Autodesk Fusion 360 part; units mm, degrees
note: some values were not read from the file. Set by a fixed rule: which sketch regions a step uses.
(part 2 of 2)
  spline S166 degree 3 poles (44.496223, -52.511943) (44.032677, -52.733983) (43.546131, -52.910026) (43.0817, -53.132067) knots 0 0 0 0 1 1 1 1
  spline S167 degree 3 poles (43.0817, -53.132067) (42.433267, -53.440805) (41.829948, -53.807926) (41.141706, -54.029969) knots 0 0 0 0 1 1 1 1
  spline S168 degree 3 poles (41.141706, -54.029969) (40.538388, -54.224586) (39.320253, -54.821711) (38.725781, -54.625323) knots 0 0 0 0 1 1 1 1
  spline S169 degree 3 poles (38.725781, -54.625323) (38.425005, -54.526245) (38.187042, -54.275896) (38.151654, -53.951235) knots 0 0 0 0 1 1 1 1
  spline S170 degree 3 poles (38.151654, -53.951235) (38.101232, -53.494766) (38.35335, -53.069259) (38.402889, -52.62429) knots 0 0 0 0 1 1 1 1
  spline S171 degree 3 poles (38.402889, -52.62429) (38.444467, -52.258052) (38.431198, -51.852892) (38.384312, -51.487539) knots 0 0 0 0 1 1 1 1
  spline S172 degree 3 poles (38.384312, -51.487539) (38.315311, -50.945261) (38.092385, -50.324251) (38.721356, -50.009323) knots 0 0 0 0 1 1 1 1
  spline S173 degree 3 poles (38.721356, -50.009323) (40.090765, -49.322849) (40.129689, -51.914817) (40.06511, -52.62429) knots 0 0 0 0 1 1 1 1
  spline S174 degree 3 poles (3.607727, -48.243602) (4.740053, -47.180274) (5.990036, -46.481417) (7.50983, -46.140834) knots 0 0 0 0 1 1 1 1
  spline S175 degree 3 poles (7.50983, -46.140834) (8.096341, -46.00991) (8.691695, -45.924101) (9.292362, -45.897561) knots 0 0 0 0 1 1 1 1
  spline S176 degree 3 poles (9.292362, -45.897561) (9.454251, -45.889599) (9.613484, -45.942678) (9.774487, -45.911715) knots 0 0 0 0 1 1 1 1
  spline S177 degree 3 poles (9.774487, -45.911715) (10.134532, -45.842714) (10.56269, -45.601209) (10.90062, -45.453477) knots 0 0 0 0 1 1 1 1
  spline S178 degree 3 poles (10.90062, -45.453477) (11.100547, -45.366782) (11.265972, -45.223473) (11.45705, -45.120855) knots 0 0 0 0 1 1 1 1
  spline S179 degree 3 poles (11.45705, -45.120855) (12.492954, -44.563539) (13.561589, -44.033647) (14.614296, -43.507291) knots 0 0 0 0 1 1 1 1
  spline S180 degree 3 poles (14.614296, -43.507291) (16.420715, -42.602313) (18.244822, -41.723876) (20.039735, -40.791474) knots 0 0 0 0 1 1 1 1
  spline S181 degree 3 poles (20.039735, -40.791474) (20.539553, -40.531393) (21.011057, -40.22089) (21.513526, -39.967884) knots 0 0 0 0 1 1 1 1
  spline S182 degree 3 poles (21.513526, -39.967884) (23.597715, -38.917828) (25.688097, -37.874851) (27.798829, -36.8761) knots 0 0 0 0 1 1 1 1
  spline S183 degree 3 poles (27.798829, -36.8761) (28.349066, -36.616018) (28.951499, -36.454135) (29.485819, -36.170167) knots 0 0 0 0 1 1 1 1
  spline S184 degree 3 poles (29.485819, -36.170167) (29.45574, -35.344805) (29.262891, -34.507063) (29.145234, -33.690546) knots 0 0 0 0 1 1 1 1
  spline S185 degree 3 poles (29.145234, -33.690546) (29.062964, -33.119078) (29.078886, -32.501608) (29.055, -31.923941) knots 0 0 0 0 1 1 1 1
  spline S186 degree 3 poles (29.055, -31.923941) (29.030233, -31.341853) (29.185928, -30.081255) (28.996616, -29.618595) knots 0 0 0 0 1 1 1 1
  spline S187 degree 3 poles (28.996616, -29.618595) (28.600304, -29.789328) (28.245566, -30.021986) (27.865176, -30.221028) knots 0 0 0 0 1 1 1 1
  spline S188 degree 3 poles (27.865176, -30.221028) (26.969045, -30.691652) (26.013646, -31.079121) (25.104243, -31.527629) knots 0 0 0 0 1 1 1 1
  spline S189 degree 3 poles (25.104243, -31.527629) (24.477038, -31.837249) (23.805606, -32.041599) (23.171328, -32.33264) knots 0 0 0 0 1 1 1 1
  spline S190 degree 3 poles (23.171328, -32.33264) (22.350389, -32.710379) (21.53122, -33.112885) (20.720016, -33.512739) knots 0 0 0 0 1 1 1 1
  spline S191 degree 3 poles (20.720016, -33.512739) (20.259121, -33.739205) (19.845115, -34.058555) (19.396607, -34.309787) knots 0 0 0 0 1 1 1 1
  spline S192 degree 3 poles (19.396607, -34.309787) (18.371323, -34.883031) (17.33719, -35.434154) (16.30925, -35.999434) knots 0 0 0 0 1 1 1 1
  spline S193 degree 3 poles (16.30925, -35.999434) (15.018572, -36.708909) (13.800435, -37.562574) (12.556645, -38.348126) knots 0 0 0 0 1 1 1 1
  spline S194 degree 3 poles (12.556645, -38.348126) (12.074526, -38.652439) (11.581786, -39.118641) (11.05543, -39.333606) knots 0 0 0 0 1 1 1 1
  spline S195 degree 3 poles (11.05543, -39.333606) (10.580384, -39.52734) (9.238401, -39.030178) (8.65012, -38.967367) knots 0 0 0 0 1 1 1 1
  spline S196 degree 3 poles (8.65012, -38.967367) (7.122362, -38.803713) (4.887785, -39.286718) (3.877539, -40.553509) knots 0 0 0 0 1 1 1 1
  spline S197 degree 3 poles (3.877539, -40.553509) (3.406915, -41.142673) (3.48034, -42.098075) (3.525457, -42.81197) knots 0 0 0 0 1 1 1 1
  spline S198 degree 3 poles (3.525457, -42.81197) (3.610384, -44.165456) (3.557303, -45.533093) (3.613035, -46.887462) knots 0 0 0 0 1 1 1 1
  spline S199 degree 3 poles (3.613035, -46.887462) (3.6325, -47.347471) (3.490956, -47.796862) (3.607727, -48.243602) knots 0 0 0 0 1 1 1 1
  spline S200 degree 3 poles (57.658637, -47.275816) (57.840871, -46.873308) (57.889526, -46.423917) (57.977105, -45.992217) knots 0 0 0 0 1 1 1 1
  spline S201 degree 3 poles (57.977105, -45.992217) (58.236301, -44.721889) (58.388457, -43.487829) (58.374303, -42.185653) knots 0 0 0 0 1 1 1 1
  spline S202 degree 3 poles (58.374303, -42.185653) (58.368995, -41.741569) (58.44242, -40.848978) (58.269917, -40.46947) knots 0 0 0 0 1 1 1 1
  spline S203 degree 3 poles (58.269917, -40.46947) (58.06999, -40.031577) (57.470211, -39.642341) (57.133167, -39.306182) knots 0 0 0 0 1 1 1 1
  spline S204 degree 3 poles (57.133167, -39.306182) (56.783737, -38.958523) (56.379463, -38.714364) (55.987569, -38.421552) knots 0 0 0 0 1 1 1 1
  spline S205 degree 3 poles (55.987569, -38.421552) (54.822513, -37.551073) (53.586684, -36.786751) (52.326086, -36.064896) knots 0 0 0 0 1 1 1 1
  spline S206 degree 3 poles (52.326086, -36.064896) (51.10618, -35.366921) (49.832313, -34.771567) (48.571715, -34.154096) knots 0 0 0 0 1 1 1 1
  spline S207 degree 3 poles (48.571715, -34.154096) (46.786532, -33.280081) (45.011078, -32.400758) (43.141854, -31.714285) knots 0 0 0 0 1 1 1 1
  spline S208 degree 3 poles (43.141854, -31.714285) (41.294745, -31.035775) (39.388368, -30.525341) (37.491721, -30.015793) knots 0 0 0 0 1 1 1 1
  spline S209 degree 3 poles (37.491721, -30.015793) (35.641958, -29.519517) (32.587333, -28.857815) (30.72076, -29.181588) knots 0 0 0 0 1 1 1 1
  spline S210 degree 3 poles (30.72076, -29.181588) (30.505795, -30.287375) (30.619911, -31.514357) (30.691566, -32.631646) knots 0 0 0 0 1 1 1 1
  spline S211 degree 3 poles (30.691566, -32.631646) (30.760569, -33.722396) (30.826031, -34.897183) (31.119729, -35.949895) knots 0 0 0 0 1 1 1 1
  spline S212 degree 3 poles (31.119729, -35.949895) (32.315751, -36.25863) (33.53654, -36.481558) (34.74052, -36.76287) knots 0 0 0 0 1 1 1 1
  spline S213 degree 3 poles (34.74052, -36.76287) (36.101967, -37.080449) (37.467837, -37.500649) (38.806283, -37.911119) knots 0 0 0 0 1 1 1 1
  spline S214 degree 3 poles (38.806283, -37.911119) (41.051472, -38.597592) (43.309933, -39.356607) (45.480817, -40.250967) knots 0 0 0 0 1 1 1 1
  spline S215 degree 3 poles (45.480817, -40.250967) (47.174883, -40.948939) (48.829143, -41.79553) (50.469248, -42.610274) knots 0 0 0 0 1 1 1 1
  spline S216 degree 3 poles (50.469248, -42.610274) (51.958079, -43.349826) (53.436296, -44.207916) (54.774742, -45.198703) knots 0 0 0 0 1 1 1 1
  spline S217 degree 3 poles (54.774742, -45.198703) (55.714219, -45.894907) (56.613889, -46.744152) (57.658637, -47.275816) knots 0 0 0 0 1 1 1 1
  spline S218 degree 3 poles (3.430801, -33.476467) (4.020848, -33.334042) (4.602051, -33.141194) (5.202718, -33.039459) knots 0 0 0 0 1 1 1 1
  spline S219 degree 3 poles (5.202718, -33.039459) (5.752956, -32.946574) (6.323543, -32.936844) (6.872015, -32.834224) knots 0 0 0 0 1 1 1 1
  spline S220 degree 3 poles (6.872015, -32.834224) (7.173672, -32.777612) (7.468255, -32.659954) (7.769026, -32.5998) knots 0 0 0 0 1 1 1 1
  spline S221 degree 3 poles (7.769026, -32.5998) (8.635083, -32.427296) (9.597561, -32.286638) (10.265456, -31.636437) knots 0 0 0 0 1 1 1 1
  spline S222 degree 3 poles (10.265456, -31.636437) (11.121777, -30.804002) (11.23147, -29.671671) (11.666707, -28.618079) knots 0 0 0 0 1 1 1 1
  spline S223 degree 3 poles (11.666707, -28.618079) (12.317799, -27.046089) (13.740281, -25.306908) (15.289269, -24.53905) knots 0 0 0 0 1 1 1 1
  spline S224 degree 3 poles (15.289269, -24.53905) (17.057644, -23.663264) (18.438556, -23.862305) (20.298931, -24.222351) knots 0 0 0 0 1 1 1 1
  spline S225 degree 3 poles (20.298931, -24.222351) (21.102177, -24.377161) (21.973535, -24.74605) (22.799782, -24.690318) knots 0 0 0 0 1 1 1 1
  spline S226 degree 3 poles (22.799782, -24.690318) (23.20671, -24.662895) (23.589756, -24.503662) (23.975454, -24.38689) knots 0 0 0 0 1 1 1 1
  spline S227 degree 3 poles (23.975454, -24.38689) (24.745083, -24.151581) (25.526213, -23.921574) (26.24984, -23.5633) knots 0 0 0 0 1 1 1 1
  spline S228 degree 3 poles (26.24984, -23.5633) (27.207896, -23.088254) (28.034138, -22.413281) (29.033769, -22.016082) knots 0 0 0 0 1 1 1 1
  spline S229 degree 3 poles (29.033769, -22.016082) (28.970078, -21.072183) (28.764844, -20.131821) (28.690532, -19.185266) knots 0 0 0 0 1 1 1 1
  spline S230 degree 3 poles (28.690532, -19.185266) (28.624185, -18.355482) (28.708226, -17.531891) (28.75688, -16.708301) knots 0 0 0 0 1 1 1 1
  spline S231 degree 3 poles (28.75688, -16.708301) (28.163296, -16.734839) (27.657285, -17.040923) (27.118548, -17.260309) knots 0 0 0 0 1 1 1 1
  spline S232 degree 3 poles (27.118548, -17.260309) (26.225068, -17.623891) (25.36521, -18.041439) (24.485887, -18.440408) knots 0 0 0 0 1 1 1 1
  spline S233 degree 3 poles (24.485887, -18.440408) (22.60074, -19.294959) (20.712937, -20.170745) (18.885293, -21.146489) knots 0 0 0 0 1 1 1 1
  spline S234 degree 3 poles (18.885293, -21.146489) (18.255437, -21.483533) (17.663619, -21.879851) (17.039956, -22.224854) knots 0 0 0 0 1 1 1 1
  spline S235 degree 3 poles (17.039956, -22.224854) (16.696719, -22.415051) (16.334017, -22.563669) (16.002281, -22.771555) knots 0 0 0 0 1 1 1 1
  spline S236 degree 3 poles (16.002281, -22.771555) (15.494504, -23.090025) (15.005306, -23.436798) (14.489565, -23.742882) knots 0 0 0 0 1 1 1 1
  spline S237 degree 3 poles (14.489565, -23.742882) (13.972939, -24.050732) (13.428894, -24.311699) (12.944999, -24.67263) knots 0 0 0 0 1 1 1 1
  spline S238 degree 3 poles (12.944999, -24.67263) (12.352296, -25.113174) (11.460592, -25.985418) (10.8095, -26.256115) knots 0 0 0 0 1 1 1 1
  spline S239 degree 3 poles (10.8095, -26.256115) (9.984144, -26.598466) (9.260517, -25.758953) (8.467886, -25.618294) knots 0 0 0 0 1 1 1 1
  spline S240 degree 3 poles (8.467886, -25.618294) (7.178094, -25.388293) (5.681301, -25.827957) (4.567549, -26.474621) knots 0 0 0 0 1 1 1 1
  spline S241 degree 3 poles (4.567549, -26.474621) (4.28093, -26.640932) (3.845693, -26.873585) (3.637807, -27.136323) knots 0 0 0 0 1 1 1 1
  spline S242 degree 3 poles (3.637807, -27.136323) (3.415764, -27.41852) (3.384799, -28.457075) (3.367991, -28.827735) knots 0 0 0 0 1 1 1 1
  spline S243 degree 3 poles (3.367991, -28.827735) (3.344995, -29.301011) (3.257412, -29.768983) (3.237067, -30.243144) knots 0 0 0 0 1 1 1 1
  spline S244 degree 3 poles (3.237067, -30.243144) (3.211415, -30.865922) (3.254761, -31.479855) (3.280413, -32.100868) knots 0 0 0 0 1 1 1 1
  spline S245 degree 3 poles (3.280413, -32.100868) (3.299878, -32.562642) (3.247682, -33.046537) (3.430801, -33.476467) knots 0 0 0 0 1 1 1 1
  spline S246 degree 3 poles (58.012489, -31.800977) (58.306187, -30.813732) (58.438882, -29.070123) (58.391111, -28.031568) knots 0 0 0 0 1 1 1 1
  spline S247 degree 3 poles (58.391111, -28.031568) (58.371649, -27.61314) (58.392881, -27.023088) (58.200031, -26.642698) knots 0 0 0 0 1 1 1 1
  spline S248 degree 3 poles (58.200031, -26.642698) (58.021336, -26.28796) (57.051782, -25.718258) (56.69793, -25.499757) knots 0 0 0 0 1 1 1 1
  spline S249 degree 3 poles (56.69793, -25.499757) (55.56118, -24.798246) (54.458046, -24.063118) (53.278832, -23.431491) knots 0 0 0 0 1 1 1 1
  spline S250 degree 3 poles (53.278832, -23.431491) (51.004448, -22.214239) (48.64337, -21.175684) (46.263715, -20.186668) knots 0 0 0 0 1 1 1 1
  spline S251 degree 3 poles (46.263715, -20.186668) (43.422283, -19.005683) (40.539273, -17.813203) (37.501453, -17.256773) knots 0 0 0 0 1 1 1 1
  spline S252 degree 3 poles (37.501453, -17.256773) (36.213429, -17.020578) (34.879408, -16.950689) (33.602001, -16.649032) knots 0 0 0 0 1 1 1 1
  spline S253 degree 3 poles (33.602001, -16.649032) (32.720908, -16.441141) (31.27631, -16.015634) (30.420869, -16.354449) knots 0 0 0 0 1 1 1 1
  spline S254 degree 3 poles (30.420869, -16.354449) (30.257214, -17.259424) (30.217405, -18.180327) (30.281987, -19.096802) knots 0 0 0 0 1 1 1 1
  spline S255 degree 3 poles (30.281987, -19.096802) (30.334177, -19.835467) (30.427062, -20.579444) (30.542948, -21.308378) knots 0 0 0 0 1 1 1 1
  spline S256 degree 3 poles (30.542948, -21.308378) (30.588065, -21.58969) (30.555334, -21.988659) (30.676528, -22.241662) knots 0 0 0 0 1 1 1 1
  spline S257 degree 3 poles (30.676528, -22.241662) (30.733146, -22.360205) (30.893264, -22.459283) (30.988805, -22.54509) knots 0 0 0 0 1 1 1 1
  spline S258 degree 3 poles (30.988805, -22.54509) (31.900859, -23.366915) (33.222497, -22.816672) (34.192048, -22.390279) knots 0 0 0 0 1 1 1 1
  spline S259 degree 3 poles (34.192048, -22.390279) (35.848079, -21.661345) (37.066214, -20.20259) (38.744358, -19.51258) knots 0 0 0 0 1 1 1 1
  spline S260 degree 3 poles (38.744358, -19.51258) (39.465331, -19.215345) (40.253537, -19.131304) (41.027588, -19.148998) knots 0 0 0 0 1 1 1 1
  spline S261 degree 3 poles (41.027588, -19.148998) (41.59729, -19.162264) (42.163453, -19.273729) (42.673884, -19.532925) knots 0 0 0 0 1 1 1 1
  spline S262 degree 3 poles (42.673884, -19.532925) (43.894675, -20.152166) (44.947385, -21.364996) (45.548932, -22.57694) knots 0 0 0 0 1 1 1 1
  spline S263 degree 3 poles (45.548932, -22.57694) (46.173484, -23.836653) (46.612259, -25.483834) (47.887012, -26.258771) knots 0 0 0 0 1 1 1 1
  spline S264 degree 3 poles (47.887012, -26.258771) (48.545177, -26.65862) (49.435998, -26.484351) (50.142819, -26.314503) knots 0 0 0 0 1 1 1 1
  spline S265 degree 3 poles (50.142819, -26.314503) (51.325569, -26.02965) (52.686131, -25.785491) (53.724686, -26.613503) knots 0 0 0 0 1 1 1 1
  spline S266 degree 3 poles (53.724686, -26.613503) (54.588086, -27.301748) (55.100285, -28.31288) (55.556755, -29.292166) knots 0 0 0 0 1 1 1 1
  spline S267 degree 3 poles (55.556755, -29.292166) (55.769068, -29.745982) (55.9628, -30.214835) (56.281267, -30.606726) knots 0 0 0 0 1 1 1 1
  spline S268 degree 3 poles (56.281267, -30.606726) (56.720929, -31.148119) (57.3039, -31.699247) (58.012489, -31.800977) knots 0 0 0 0 1 1 1 1
extrude "Extrude19" cut sketch "Sketch11" against normal blind 0.4 contours S0 S1 S2 S3 S4 S5 S6 S7 S8 S9 S10 S11 S12 S13 S14 S15 S16 S17 S18 S19 S20 S21 S22 S23 S24 S25 S26 S27 S28 S29 S30 S31 S32 S33 S34 S35 S36 S37 S38 S39 S40 S41 S42 S43 S44 S45 S46 S47 S48 S49 S50 S51 S52 S53 S54 S55 | S93 S94 S95 S96 S97 S98 S99 S100 S101 S102 S103 S104 S105 S106 S107 S108 S109 S110 S111 S112 S113 S114 | S115 S116 S117 S118 S119 S120 S121 S122 S123 S124 S125 S126 S127 S128 S129 S130 S131 S132 S133 S134 S135 S136 S137 S138 S139 S140 S141 | S142 S143 S144 S145 S146 S147 S148 S149 S150 S151 S152 S153 S154 S155 S156 S157 S158 S159 S160 S161 S162 S163 S164 S165 S166 S167 S168 S169 S170 S171 S172 S173 picked at (39.975888, -24.403827) picked at (34.820138, -52.560596) picked at (19.619316, -48.541536) picked at (45.37702, -50.765682) bodies 1
fillet "Fillet2" radius 1.5 8 edges at (62.635534, 81.635534, 21.3) (30.9, 83.1, 21.3) (-0.835534, 81.635534, 21.3) (-2.3, 40.4, 21.3) (-0.835534, -0.835534, 21.3) (30.9, -2.3, 21.3) (62.635534, -0.835534, 21.3) (64.1, 40.4, 21.3) on bodies 2
fillet "Fillet3" radius 1.5 8 edges at (64.1, 40.4, 0) (62.635534, 81.635534, 0) (30.9, 83.1, 0) (-0.835534, 81.635534, 0) (-2.3, 40.4, 0) (-0.835534, -0.835534, 0) (30.9, -2.3, 0) (62.635534, -0.835534, 0) on bodies 1
equation "d8 = 12 mm + 1.5 mm"
equation "d10 = 12 mm + 1.5 mm + 6.3 mm"
equation "d28 = thick"
equation "d30 = thick"
equation "d31 = thick"
equation "d45 = -1.5 mm - 4 mm"
equation "d75 = ( 12 / 2 ) * 1 mm"
equation "d76 = ( 12 / 2 ) * 1 mm"
equation "d84 = 8.3 mm - 2.5 mm"
equation "d91 = space"
equation "d94 = space"
equation "d107 = space"
equation "d108 = space"
equation "d109 = tol"
equation "d110 = tol"
equation "d111 = tol"
equation "d112 = tol"
equation "d113 = tol"
equation "d114 = tol"
equation "d115 = tol"
equation "d116 = tol"
equation "d117 = tol"
equation "tol = -0.7 mm"
equation "space = 3.5 mm"
equation "d153 = thick"
equation "thick = 2.3 mm"
